Autodesk Inventor part; units mm, degrees
(part 2 of 2)
  point P139 (21.25, -57.5)
  point P140 (20.3012, -58.3139)
  point P141 (22.0883, -60.3972)
  point P142 (17.8726, -60.3972)
  point P143 (16.6119, -68.5849)
  point P144 (20.8276, -68.5849)
  point P145 (24.2412, -46.4151)
  point P146 (20.0255, -46.4151)
  point P147 (22.9805, -54.6028)
  point P148 (18.7648, -54.6028)
  point P149 (30.7588, -68.5849)
  point P150 (32.0195, -60.3972)
  point P151 (32.5459, -70.6683)
  point P152 (34.9745, -68.5849)
  point P153 (34.1158, -41.4346)
  point P154 (29.81, -69.3988)
  point P155 (21.5258, -69.3988)
  point P156 (29.1684, -73.5654)
  point P157 (31.5971, -71.4821)
  point P158 (20.8842, -73.5654)
  point P159 (19.0971, -71.4821)
  point P160 (18.399, -70.6683)
  point P161 (25.8316, -41.4346)
  point P162 (27.5, -57.5)
  point P163 (19.8269, -58.7208)
  point P164 (35.496, -43.0435)
  point P165 (29.9971, -69.6169)
  point P166 (21.3502, -69.5494)
  dimension "d24" = 1.25
  dimension "d25" = 4.1667
  dimension "d26" = 4.1667
  dimension "d27" = 12.5
  dimension "d28" = 12.5
  dimension "d29" = 0.625
  dimension "d30" = 14.1469
  dimension "d31" = 14.1469
  dimension "d32" = 14.1469
  dimension "d33" = 20
  dimension "d34" = 20
  dimension "d36" = 22.5
  dimension "d37" = 8
  constraints: 364 end point, 337 point on line, 336 point on circle, 168 centre point, 24 tangent, 11 equal radius, 8 collinear, 8 midpoint, 5 parallel, 4 coincident, 4 horizontal, 2 vertical alignment, 1 perpendicular, 961 other
  measures "d24" distance between parallel lines of L18 L21
  measures "d25" distance between parallel lines of L17 L24
  measures "d26" distance between parallel lines of L13 L12
  measures "d27" distance of L22.start L22.end
  measures "d28" distance of L20.start L20.end
  measures "d29" radius of A22
  measures "d30" distance of L18.start L42.start
  measures "d31" distance of L18.start L6.start
  measures "d32" distance of L24.start L2.start
  measures "d33" distance of point (23.679, -55.417) point (3.679, -55.417)
  measures "d34" distance of point (23.679, -55.417) point (43.679, -55.417)
  measures "d36" distance of L182.start point (27.5, -57.5)
  measures "d37" angle of L3 L182
extrude "Extrusion2" cut sketch "Sketch2" along normal blind 33 contours L12 L13 E2 L8 E6 A0 E1 L1 E0
sketch "Sketch4" plane through (16.25, 0, 100) normal (0, 0, 1) x (1, 0, 0)
  line L0 (-8.75, -14.15) -> (31.25, -14.15) construction
  line L1 (31.25, -14.15) -> (31.25, 14.15) construction
  line L2 (31.25, 14.15) -> (-8.75, 14.15) construction
  line L3 (-8.75, 14.15) -> (-8.75, -14.15) construction
  line L4 (0, 0) -> (22.5, 0) projected
  line L5 (-8.75, -14.15) -> (31.25, 14.15) construction
  line L6 (31.25, -14.15) -> (-8.75, 14.15) construction
  line L7 (57, 0) -> (22.5, 0) projected
  arc A0 (17.1, -12.15) -> (17.1, 12.15) centre (17.1, 0) ccw
  line L8 (17.1, 12.15) -> (5.4, 12.15)
  line L9 (11.25, 14.15) -> (11.25, -14.15) construction
  arc A1 (5.4, 12.15) -> (5.4, -12.15) centre (5.4, 0) ccw
  line L10 (17.1, -12.15) -> (5.4, -12.15)
  point P0 (-16.25, 0)
  point P1 (11.25, 0)
  point P2 (55.2949, 0)
  point P3 (29.25, 0)
  point P4 (31.25, 0)
  point P5 (5.4, -12.15)
  dimension "d44" = 40
  dimension "d45" = 28.3
  dimension "d50" = 2
  dimension "d51" = 2
  constraints: 18 end point, 6 midpoint, 5 point on circle, 5 symmetric about line, 2 centre point, 2 horizontal, 2 parallel, 1 perpendicular, 1 point on line, 1 tangent, 1 other
  measures "d44" distance of L2.end L1.end
  measures "d45" distance of L1.end L0.end
  measures "d50" distance of point (29.25, 0) point (31.25, 0)
  measures "d51" distance from line of L2 L8.start
extrude "Extrusion3" cut sketch "Sketch4" against normal blind 5
fillet "R2" radius 2 2 edges at (39, 16.5, 34.7671) (71.4285, 16.5, 67.1956)
mirror "Mirror1" about plane through (0, 0, 0) normal (0, 1, 0)
extrude "Extrusion4" cut sketch "Sketch3" against normal blind 0.5 contours L6 A1 L28 A34 L35 A28 L36 A35 L26 A18 L39 A33 | L7 A4 L16 A13 L14 A15 L19 A37 L42 A9 L8 A3 | L9 A6 L43 A41 L44 A26 L32 A25 L31 A11 L29 A5 | L11 A8 L27 A10 L12 A14 L25 A22 L18 A17 L13 A7 | A19 L21 A20 L23 A21 L24 A39 L45 A38 L41 A40 L17 | L30 A30 L38 A31 L37 A29 L34 A32 L33 A27 L40 A23 | L48 A57 L70 A59 L71 A62 L49 A48 L56 A55 L68 A53 | L61 A82 L91 A81 L90 A66 L78 A67 L79 A69 L52 A42 | L55 A64 L76 A76 L75 A74 L74 A61 L73 A63 L77 A46 | L64 A54 L67 A56 L72 A60 L66 A52 L63 A83 L62 A51 | L81 A72 L83 A73 L82 A71 L84 A77 L85 A75 L86 A70 | L93 A99 L115 A101 L116 A104 L94 A90 L101 A97 L113 A95 | L106 A124 L136 A123 L135 A108 L123 A109 L124 A111 L97 A84 | A85 L98 A110 L125 A107 L96 A86 L99 A87 L114 A100 L95 | L102 A89 L105 A120 L132 A121 L133 A122 L104 A92 L103 A91 | L126 A114 L128 A115 L127 A113 L129 A119 L130 A117 L131 A112 | L188 S0 S1 S2 L189 S3 S4 S5 S6 L190 S7 S8 S9 S10 S11 S12 L191 | L192 L193 S13 S14 S15 L194 L195 L196 S16 S17 S18 S19 L197 | L198 S20 S21 S22 L199 S23 S24 S25 S26 L200 S27 S28 S29 S30 S31 S32 L201 | L202 L203 L204 L205 L206 L207 L208 L209 | L210 L211 L212 L213 L214 L215 L216 L217 | L221 L222 L223 L224 L225 L226 L227 L228 L229 L230 L231 L232 | L233 L234 L235 L236 L237 L238 L239 L240 L241 L242 | L243 L244 L245 L246 L247 L248 L249 L250 | L254 L255 L256 L257 | S33 S34 S35 S36 | L258 L259 L260 L261 S42 S43 S44 S45 L262
pattern_circular "Circular Pattern1" count 2 over 360 about axis through (27.5, 0, 100) along (0, 0, 1) of "Extrusion4"
equation "\"d4\" = d1"
equation "\"d5\" = d1"
equation "\"d52\" = d1"
equation "\"d34\" = d33"
equation "\"d51\" = d50"
equation "\"d24\" = 0.1 * d27"
equation "\"d25\" = 0.333333 * d27"
equation "\"d26\" = d25"
equation "\"d28\" = d27"
equation "\"d29\" = 0.05 * d27"
body "Solid1"
